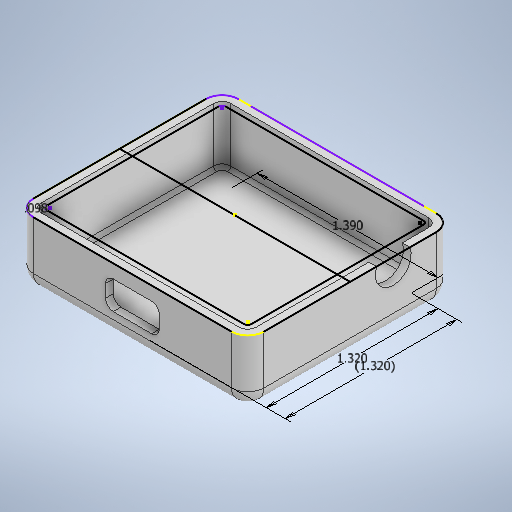
# Autodesk Inventor part: calendate
Saved by Autodesk Inventor 2025 (Build 290162000, 162)
## iProperties
Created: 2026-06-17
Part Number: calendate
Material: Generic
Document SubType Name: Modeling
Designer: dalto
Density: 1 g/cm^3
Appearance: Default
Author: dalto
Autodesk Inventor part; units mm, degrees
ref_plane "YZ Plane" through (0, 0, 0) normal (1, 0, 0) x (0, 1, 0)
ref_plane "XZ Plane" through (0, 0, 0) normal (0, 1, 0) x (-1, 0, 0)
ref_plane "XY Plane" through (0, 0, 0) normal (0, 0, 1) x (1, 0, 0)
sketch "Sketch1" plane through (0, 0, 0) normal (0, 1, 0) x (-1, 0, 0)
  line L0 (-22.5, 20) -> (22.5, 20)
  line L1 (22.5, 20) -> (22.5, -20)
  line L2 (22.5, -20) -> (-22.5, -20)
  line L3 (-22.5, -20) -> (-22.5, 20)
  line L4 (-22.5, 20) -> (22.5, -20) construction
  line L5 (22.5, 20) -> (-22.5, -20) construction
  point P0 (0, 0)
  dimension "d0" = 45
  dimension "d1" = 40
  constraints: 12 end point, 2 midpoint, 2 parallel, 1 horizontal, 1 perpendicular
  measures "d0" distance of L1.end L2.end
  measures "d1" distance of L0.end L1.end
extrude "Extrusion1" add sketch "Sketch1" along normal blind 12.7
fillet "Fillet1" radius 3.175 4 edges at (22.5, 6.35, 20) (22.5, 6.35, -20) (-22.5, 6.35, -20) (-22.5, 6.35, 20)
sketch "Sketch2" plane through (0, 12.7, 0) normal (0, 1, 0) x (1, 0, 0)
  line L0 (-22.5, 16.825) -> (-22.5, -16.825) projected
  line L1 (-22.5, 16.825) -> (-22.5, -16.825)
  arc A0 (-22.5, -16.825) -> (-19.325, -20) centre (-19.325, -16.825) ccw
  line L2 (-19.325, -20) -> (19.325, -20)
  arc A1 (19.325, -20) -> (22.5, -16.825) centre (19.325, -16.825) ccw projected
  line L3 (22.5, -16.825) -> (22.5, 16.825)
  line L4 (-22.5, 0) -> (22.5, 0)
  arc A2 (-19.325, 20) -> (-22.5, 16.825) centre (-19.325, 16.825) ccw
  arc A3 (22.5, 16.825) -> (19.325, 20) centre (19.325, 16.825) ccw
  line L5 (-16.825, 20) -> (16.825, 20)
  line L6 (19.325, 20) -> (-19.325, 20) projected
  arc A4 (-20, -16.825) -> (-19.325, -17.5) centre (-19.325, -16.825) ccw
  line L7 (-20, -16.825) -> (-20, 16.825)
  arc A5 (-19.325, 17.5) -> (-20, 16.825) centre (-19.325, 16.825) ccw
  line L8 (-19.325, 17.5) -> (19.325, 17.5)
  arc A6 (20, 16.825) -> (19.325, 17.5) centre (19.325, 16.825) ccw
  line L9 (20, 16.825) -> (20, -16.825)
  arc A7 (19.325, -17.5) -> (20, -16.825) centre (19.325, -16.825) ccw
  line L10 (19.325, -17.5) -> (-19.325, -17.5)
  point P0 (0, 0)
  dimension "d28" = 2.5
  constraints: 18 end point, 16 point on circle, 7 centre point, 4 symmetric about line, 2 midpoint, 2 vertical, 1 horizontal, 1 point on line, 1 tangent, 9 other
  measures "d28" radial gap between concentric circles of A0 A4
shell "Shell1" thickness 1.5 removed faces 1 at (-6.4417, 12.7, -6.6667)
fillet "Fillet2" radius 0.635 8 edges at (-20.5094, 1.5, 18.0094) (0, 1.5, 18.5) (20.5094, 1.5, 18.0094) (21, 1.5, 0) (20.5094, 1.5, -18.0094) (0, 1.5, -18.5) (-20.5094, 1.5, -18.0094) (-21, 1.5, 0)
sketch "Sketch3" plane through (22.5, 0, 16.825) normal (1, 0, 0) x (0, 0, -1)
  line L0 (33.65, 12.7) -> (0, 12.7) projected
  line L1 (33.65, 12.7) -> (33.65, -12.7)
  line L2 (16.825, 12.7) -> (16.825, 0)
  line L3 (33.65, 12.7) -> (16.825, 12.7)
  line L4 (25.2375, 12.7) -> (25.2375, 10.1)
  circle A0 centre (25.2375, 11.4) radius 3.5
  line L5 (0, 2.135) -> (33.65, 2.135) projected
  line L6 (25.2375, 2.135) -> (25.2375, -2.565)
  dimension "d8" = 7
  constraints: 10 end point, 3 midpoint, 3 vertical, 2 point on line, 1 centre point, 1 collinear
  measures "d8" diameter of A0
extrude "Extrusion2" cut sketch "Sketch3" against normal blind 7 contours A0 L0 | L0 A0
fillet "Fillet4" radius 3.175 8 edges at (21.5701, 0, 19.0701) (22.5, 0, 0) (21.5701, 0, -19.0701) (0, 0, -20) (-21.5701, 0, -19.0701) (-22.5, 0, 0) (-21.5701, 0, 19.0701) (0, 0, 20)
sketch "Sketch5" plane through (19.325, 12.7, 18.5) normal (0, 0, -1) x (-1, 0, 0)
  line L0 (38.65, -10.565) -> (38.65, 0) projected
  line L1 (38.65, -5.2825) -> (38.65, -3.7825)
  line L2 (38.65, 0) -> (0, 0) projected
  line L3 (9.1307, 0) -> (9.1307, 6.35)
  line L4 (9.1307, 0) -> (15.4807, 0) construction
  line L5 (9.1307, 6.35) -> (9.1307, 0)
  line L6 (6.35, 6.35) -> (6.35, 0.35)
  line L7 (6.35, 0.35) -> (6.35, -2.65)
  line L8 (6.35, -2.65) -> (19.325, -2.65)
  line L9 (19.325, -2.65) -> (19.325, -5.4)
  line L10 (14.075, -8.15) -> (24.575, -8.15)
  line L11 (24.575, -8.15) -> (24.575, -2.65)
  line L12 (24.575, -2.65) -> (14.075, -2.65)
  line L13 (14.075, -2.65) -> (14.075, -8.15)
  line L14 (14.075, -8.15) -> (24.575, -2.65) construction
  line L15 (24.575, -8.15) -> (14.075, -2.65) construction
  point P0 (19.325, -12.7)
  point P1 (14.075, -2.65)
  dimension "d45" = 90
  dimension "d46" = 6.35
  dimension "d47" = 6
  dimension "d49" = 3
  dimension "d50" = 2.75
  dimension "d51" = 10.5
  dimension "d52" = 5.5
  constraints: 28 end point, 3 midpoint, 3 parallel, 3 perpendicular, 3 point on line, 2 horizontal, 2 vertical
  measures "d45" angle of L4 L3
  measures "d46" distance of L3.end L5.end
  measures "d47" distance of L6.start L6.end
  measures "d49" distance of L6.end L7.end
  measures "d50" distance of L8.end L9.end
  measures "d51" distance of L12.end L11.end
  measures "d52" distance of L11.end L10.end
extrude "Extrusion6" cut sketch "Sketch5" against normal blind 12.7
fillet "Fillet5" radius 1.5 4 edges at (-5.25, 10.05, 19.25) (5.25, 10.05, 19.25) (5.25, 4.55, 19.25) (-5.25, 4.55, 19.25)
sketch "Sketch6" plane through (0, 0, 0) normal (0, -1, 0) x (1, 0, 0)
  line L0 (-17.653, 16.764) -> (17.653, 16.764)
  line L1 (17.653, 16.764) -> (17.653, -16.764)
  line L2 (17.653, -16.764) -> (-17.653, -16.764)
  line L3 (-17.653, -16.764) -> (-17.653, 16.764)
  line L4 (-17.653, 16.764) -> (17.653, -16.764) construction
  line L5 (17.653, 16.764) -> (-17.653, -16.764) construction
  point P0 (0, 0)
  point P1 (0, 16.764)
  dimension "d56" = 35.306
  dimension "d57" = 33.528
  dimension "d60" = 33.528
  constraints: 12 end point, 3 midpoint, 2 parallel, 1 horizontal, 1 perpendicular
  measures "d56" distance of L1.end L2.end
  measures "d57" distance of L0.end L1.end
  measures "d60" distance from line of point (0, 16.764) L2
equation "\"d9\" = d8"
body "Solid1"
